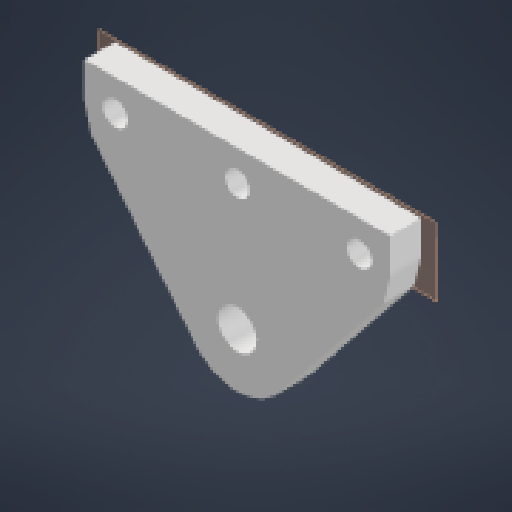
# Autodesk Inventor part: slider_02
Saved by Autodesk Inventor 2026 (Build 300175000, 175)
## iProperties
Created: 2025-12-05
Part Number: slider_02
Material: Generic
Document SubType Name: Modeling
Designer: numai
Density: 1 g/cm^3
Appearance: Default
Author: numai
Autodesk Inventor part; units mm, degrees
ref_plane "YZ Plane" through (0, 0, 0) normal (1, 0, 0) x (0, 1, 0)
ref_plane "XZ Plane" through (0, 0, 0) normal (0, 1, 0) x (-1, 0, 0)
ref_plane "XY Plane" through (0, 0, 0) normal (0, 0, 1) x (1, 0, 0)
ref_plane "作業平面1" through (-0.0753, -0.0002, 0) normal (0, 0, 1) x (1, 0.0046, 0)
sketch "スケッチ1" plane through (-0.0753, -0.0002, 0) normal (0, 0, 1) x (1, 0.0046, 0)
  line L0 (19.883, 3.9087) -> (-19.6956, 4.0909) projected
  circle A0 centre (-15.7141, 0.0725) radius 1.25 construction
  circle A1 centre (0.0753, -0.0002) radius 1.25 construction
  circle A2 centre (15.8646, -0.0729) radius 1.25 construction
  circle A3 centre (0, -16.35) radius 2.5 projected
  circle A4 centre (0, -16.35) radius 7
  line L1 (18.9963, -4.0873) -> (5.4306, -20.7668)
  line L2 (-5.4711, -20.7166) -> (-18.8826, -3.9129)
  circle A5 centre (15.8646, -0.0729) radius 1.6
  circle A6 centre (0.0753, -0.0002) radius 1.6
  circle A7 centre (-15.7141, 0.0725) radius 1.6
  line L3 (-19.6069, -0.8472) -> (-18.8826, -3.9129) projected
  line L4 (-18.8826, -3.9129) -> (18.9963, -4.0873) projected
  line L5 (18.9963, -4.0873) -> (19.7488, -1.0284) projected
  arc A8 (19.7488, -1.0284) -> (19.8645, -0.0913) centre (15.8646, -0.0729) ccw projected
  line L6 (19.8645, -0.0913) -> (19.883, 3.9087) projected
  line L7 (-19.6956, 4.0909) -> (-19.714, 0.0909) projected
  arc A9 (-19.714, 0.0909) -> (-19.6069, -0.8472) centre (-15.7141, 0.0725) ccw projected
  point P0 (0.0753, -0.0002)
  dimension "d0" = 14
  dimension "d1" = 3.2
  constraints: 4 centre point, 4 coincident, 4 end point, 2 equal radius, 2 point on circle, 2 tangent
  measures "d0" diameter of A4
  measures "d1" diameter of A5
extrude "押し出し1" add sketch "スケッチ1" along normal blind 4
sketch "スケッチ2" plane through (-0.0753, -0.0002, 0) normal (0, 0, -1) x (-1, -0.0046, 0)
  circle A0 centre (0, -16.35) radius 2.5 projected
  circle A1 centre (0, -16.35) radius 4
  point P0 (-0.0753, -0.0002)
  dimension "d4" = 8
  constraints: 1 centre point, 1 coincident
  measures "d4" diameter of A1
extrude "押し出し2" add sketch "スケッチ2" along normal blind 1
chamfer "面取り1" distance 1 angle 45 1 edges at (4, -16.3316, 0)
